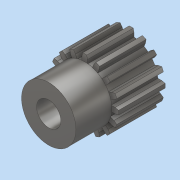
# Autodesk Inventor part: smallIdlerPinion
Saved by Autodesk Inventor 2017 (Build 210142000, 142)
## iProperties
Created: 2016-11-30
Part Number: smallIdlerPinion
Material: Steel, Carbon
Document SubType Name: Modeling
Designer: techn
Density: 7.85 g/cm^3
Appearance: Semi-Polished
Author: techn
Comments: 16 Tooth Traxxas Pinion Gear
Autodesk Inventor part; units mm, degrees
ref_plane "YZ Plane" through (0, 0, 0) normal (1, 0, 0) x (0, 1, 0)
ref_plane "XZ Plane" through (0, 0, 0) normal (0, 1, 0) x (-1, 0, 0)
ref_plane "XY Plane" through (0, 0, 0) normal (0, 0, 1) x (1, 0, 0)
sketch "Sketch1" plane through (0, 0, 0) normal (0, 0, 1) x (1, 0, 0)
  circle A0 centre (0, 0) radius 4.445
  dimension "d0" = 8.89
  constraints: 1 centre point, 1 coincident
  measures "d0" diameter of A0
extrude "Extrusion1" add sketch "Sketch1" along normal blind 6.096
sketch "Sketch2" plane through (0, 0, 6.096) normal (0, 0, 1) x (1, 0, 0)
  circle A0 centre (0, 0) radius 3.556
  dimension "d3" = 7.112
  constraints: 1 centre point, 1 coincident
  measures "d3" diameter of A0
extrude "Extrusion2" add sketch "Sketch2" along normal blind 4.699
sketch "Sketch3" plane through (0, 0, 10.795) normal (0, 0, 1) x (1, 0, 0)
  circle A0 centre (0, 0) radius 1.5875
  dimension "d6" = 3.175
  constraints: 1 centre point, 1 coincident
  measures "d6" diameter of A0
extrude "Extrusion3" cut sketch "Sketch3" against normal blind 25.4
sketch "Sketch4" plane through (0, 0, 0) normal (0, 0, -1) x (-1, 0, 0)
  circle A0 centre (0, 0) radius 3.4925
  line L0 (0.3624, 3.4737) -> (0.3624, 3.9817)
  line L1 (-0.3624, 3.4737) -> (-0.3624, 3.9817)
  line L2 (-0.3624, 3.9817) -> (-0.2617, 4.445)
  line L3 (-0.2617, 4.445) -> (0.2617, 4.445)
  line L4 (0.2617, 4.445) -> (0.3624, 3.9817)
  line L5 (-0.3624, 3.4737) -> (0.3624, 3.4737)
  line L6 (-1.6641, 3.0706) -> (-1.8585, 3.5399)
  line L7 (-1.8585, 3.5399) -> (-1.9428, 4.0065)
  line L8 (-1.9428, 4.0065) -> (-1.4592, 4.2068)
  line L9 (-1.4592, 4.2068) -> (-1.1889, 3.8172)
  line L10 (-0.9945, 3.3479) -> (-1.1889, 3.8172)
  line L11 (-1.6641, 3.0706) -> (-0.9945, 3.3479)
  line L12 (-2.7125, 2.2) -> (-3.0717, 2.5592)
  line L13 (-3.0717, 2.5592) -> (-3.3281, 2.958)
  line L14 (-3.3281, 2.958) -> (-2.958, 3.3281)
  line L15 (-2.958, 3.3281) -> (-2.5592, 3.0717)
  line L16 (-2.2, 2.7125) -> (-2.5592, 3.0717)
  line L17 (-2.7125, 2.2) -> (-2.2, 2.7125)
  line L18 (-3.3479, 0.9945) -> (-3.8172, 1.1889)
  line L19 (-3.8172, 1.1889) -> (-4.2068, 1.4592)
  line L20 (-4.2068, 1.4592) -> (-4.0065, 1.9428)
  line L21 (-4.0065, 1.9428) -> (-3.5399, 1.8585)
  line L22 (-3.0706, 1.6641) -> (-3.5399, 1.8585)
  line L23 (-3.3479, 0.9945) -> (-3.0706, 1.6641)
  line L24 (-3.4737, -0.3624) -> (-3.9817, -0.3624)
  line L25 (-3.9817, -0.3624) -> (-4.445, -0.2617)
  line L26 (-4.445, -0.2617) -> (-4.445, 0.2617)
  line L27 (-4.445, 0.2617) -> (-3.9817, 0.3624)
  line L28 (-3.4737, 0.3624) -> (-3.9817, 0.3624)
  line L29 (-3.4737, -0.3624) -> (-3.4737, 0.3624)
  line L30 (-3.0706, -1.6641) -> (-3.5399, -1.8585)
  line L31 (-3.5399, -1.8585) -> (-4.0065, -1.9428)
  line L32 (-4.0065, -1.9428) -> (-4.2068, -1.4592)
  line L33 (-4.2068, -1.4592) -> (-3.8172, -1.1889)
  line L34 (-3.3479, -0.9945) -> (-3.8172, -1.1889)
  line L35 (-3.0706, -1.6641) -> (-3.3479, -0.9945)
  line L36 (-2.2, -2.7125) -> (-2.5592, -3.0717)
  line L37 (-2.5592, -3.0717) -> (-2.958, -3.3281)
  line L38 (-2.958, -3.3281) -> (-3.3281, -2.958)
  line L39 (-3.3281, -2.958) -> (-3.0717, -2.5592)
  line L40 (-2.7125, -2.2) -> (-3.0717, -2.5592)
  line L41 (-2.2, -2.7125) -> (-2.7125, -2.2)
  line L42 (-0.9945, -3.3479) -> (-1.1889, -3.8172)
  line L43 (-1.1889, -3.8172) -> (-1.4592, -4.2068)
  line L44 (-1.4592, -4.2068) -> (-1.9428, -4.0065)
  line L45 (-1.9428, -4.0065) -> (-1.8585, -3.5399)
  line L46 (-1.6641, -3.0706) -> (-1.8585, -3.5399)
  line L47 (-0.9945, -3.3479) -> (-1.6641, -3.0706)
  line L48 (0.3624, -3.4737) -> (0.3624, -3.9817)
  line L49 (0.3624, -3.9817) -> (0.2617, -4.445)
  line L50 (0.2617, -4.445) -> (-0.2617, -4.445)
  line L51 (-0.2617, -4.445) -> (-0.3624, -3.9817)
  line L52 (-0.3624, -3.4737) -> (-0.3624, -3.9817)
  line L53 (0.3624, -3.4737) -> (-0.3624, -3.4737)
  line L54 (1.6641, -3.0706) -> (1.8585, -3.5399)
  line L55 (1.8585, -3.5399) -> (1.9428, -4.0065)
  line L56 (1.9428, -4.0065) -> (1.4592, -4.2068)
  line L57 (1.4592, -4.2068) -> (1.1889, -3.8172)
  line L58 (0.9945, -3.3479) -> (1.1889, -3.8172)
  line L59 (1.6641, -3.0706) -> (0.9945, -3.3479)
  line L60 (2.7125, -2.2) -> (3.0717, -2.5592)
  line L61 (3.0717, -2.5592) -> (3.3281, -2.958)
  line L62 (3.3281, -2.958) -> (2.958, -3.3281)
  line L63 (2.958, -3.3281) -> (2.5592, -3.0717)
  line L64 (2.2, -2.7125) -> (2.5592, -3.0717)
  line L65 (2.7125, -2.2) -> (2.2, -2.7125)
  line L66 (3.3479, -0.9945) -> (3.8172, -1.1889)
  line L67 (3.8172, -1.1889) -> (4.2068, -1.4592)
  line L68 (4.2068, -1.4592) -> (4.0065, -1.9428)
  line L69 (4.0065, -1.9428) -> (3.5399, -1.8585)
  line L70 (3.0706, -1.6641) -> (3.5399, -1.8585)
  line L71 (3.3479, -0.9945) -> (3.0706, -1.6641)
  line L72 (3.4737, 0.3624) -> (3.9817, 0.3624)
  line L73 (3.9817, 0.3624) -> (4.445, 0.2617)
  line L74 (4.445, 0.2617) -> (4.445, -0.2617)
  line L75 (4.445, -0.2617) -> (3.9817, -0.3624)
  line L76 (3.4737, -0.3624) -> (3.9817, -0.3624)
  line L77 (3.4737, 0.3624) -> (3.4737, -0.3624)
  line L78 (3.0706, 1.6641) -> (3.5399, 1.8585)
  line L79 (3.5399, 1.8585) -> (4.0065, 1.9428)
  line L80 (4.0065, 1.9428) -> (4.2068, 1.4592)
  line L81 (4.2068, 1.4592) -> (3.8172, 1.1889)
  line L82 (3.3479, 0.9945) -> (3.8172, 1.1889)
  line L83 (3.0706, 1.6641) -> (3.3479, 0.9945)
  line L84 (2.2, 2.7125) -> (2.5592, 3.0717)
  line L85 (2.5592, 3.0717) -> (2.958, 3.3281)
  line L86 (2.958, 3.3281) -> (3.3281, 2.958)
  line L87 (3.3281, 2.958) -> (3.0717, 2.5592)
  line L88 (2.7125, 2.2) -> (3.0717, 2.5592)
  line L89 (2.2, 2.7125) -> (2.7125, 2.2)
  line L90 (0.9945, 3.3479) -> (1.1889, 3.8172)
  line L91 (1.1889, 3.8172) -> (1.4592, 4.2068)
  line L92 (1.4592, 4.2068) -> (1.9428, 4.0065)
  line L93 (1.9428, 4.0065) -> (1.8585, 3.5399)
  line L94 (1.6641, 3.0706) -> (1.8585, 3.5399)
  line L95 (0.9945, 3.3479) -> (1.6641, 3.0706)
  circle A1 centre (0, 0) radius 4.7556
  dimension "d9" = 6.985
  dimension "d10" = 0.508
  dimension "d13" = 360
  dimension "d15" = 4.445
  dimension "d20" = 0.5234
  dimension "d21" = 0.7247
  dimension "d22" = 0.9714
  constraints: 192 end point, 2 centre point, 2 coincident, 2 equal length, 2 point on circle, 2 vertical, 1 horizontal, 1 perpendicular, 193 other
  measures "d9" diameter of A0
  measures "d10" distance of L0.start L0.end
  measures "d15" distance from line of L3 point (0, 0)
  measures "d20" distance of L2.end L3.end
  measures "d21" distance of L1.start L0.start
  measures "d22" distance between parallel lines of L5 L3
extrude "Extrusion4" cut sketch "Sketch4" against normal up to surface (6.096 mm away)
body "Solid1"
